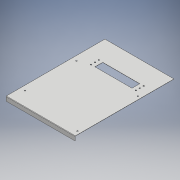
# Autodesk Inventor part: dads trunk
Saved by Autodesk Inventor 2018 (Build 220112000, 112)
## iProperties
Created: 2018-06-19
Part Number: dads trunk
Material: Generic
Document SubType Name: Sheet Metal
Designer: John Viljoen
Density: 1 g/cm^3
Flat Pattern Width: 26.3891 cm
Flat Pattern Length: 17.7174 cm
Flat Pattern Area: 467.546 cm^2
Sheet Metal Rule: Default_mm
Sheet Metal Width: 263.891 mm
Sheet Metal Length: 177.174 mm
Sheet Metal Area: 46754.619 mm^2
Appearance: Default
Author: John Viljoen
Autodesk Inventor part; units mm, degrees
ref_plane "YZ Plane" through (0, 0, 0) normal (1, 0, 0) x (0, 1, 0)
ref_plane "XZ Plane" through (0, 0, 0) normal (0, 1, 0) x (-1, 0, 0)
ref_plane "XY Plane" through (0, 0, 0) normal (0, 0, 1) x (1, 0, 0)
sketch "Sketch1" plane through (0, 0, 0) normal (0, 0, 1) x (1, 0, 0)
  line L0 (0, 0) -> (181.174, 0)
  line L1 (181.174, 0) -> (181.174, 253.26)
  line L2 (181.174, 253.26) -> (0, 253.26)
  line L3 (0, 253.26) -> (0, 0)
  dimension "d0" = 181.174
  dimension "d1" = 253.26
  measures "d0" distance of L2.end L1.end
  measures "d1" distance of L1.end L0.end
extrude "Plate1" add sketch "Sketch1" along normal blind 0.5
sketch "Sketch3" plane through (0, 0, 0.5) normal (0, 0, 1) x (1, 0, 0)
  line L0 (181.174, 253.26) -> (181.174, 0) projected
  line L1 (181.174, 253.26) -> (181.174, 168.36) construction
  line L2 (181.174, 168.36) -> (169.327, 168.36) construction
  line L3 (169.327, 168.36) -> (11.847, 168.36) construction
  line L4 (169.327, 168.36) -> (169.327, 13.48) construction
  circle A0 centre (169.327, 13.48) radius 1.5
  circle A1 centre (169.327, 168.36) radius 1.5
  circle A2 centre (11.847, 168.36) radius 1.5
  point P0 (181.174, 0.5)
  point P1 (0, 0)
  dimension "d13" = 84.9
  dimension "d14" = 11.847
  dimension "d15" = 157.48
  dimension "d16" = 154.88
  dimension "d17" = 3
  dimension "d18" = 3
  dimension "d19" = 3
  constraints: 8 end point, 3 centre point, 3 coincident, 1 horizontal, 1 perpendicular, 1 point on line, 1 vertical
  measures "d13" distance of L0.start L1.end
  measures "d14" distance of L1.end L2.end
  measures "d15" distance of L2.end L3.end
  measures "d16" distance of L2.end L4.end
  measures "d17" diameter of A0
  measures "d18" diameter of A1
  measures "d19" diameter of A2
extrude "Extrusion1" cut sketch "Sketch3" against normal blind 10
sketch "Sketch5" plane through (0, 0, 0.5) normal (0, 0, 1) x (1, 0, 0)
  circle A0 centre (11.847, 168.36) radius 1.5 projected
  line L0 (11.847, 168.36) -> (11.847, 35.808) construction
  line L1 (11.847, 168.36) -> (144.399, 168.36) construction
  line L2 (11.847, 35.808) -> (11.847, 36.34) construction
  circle A1 centre (11.847, 36.34) radius 1.5
  point P0 (0, 0)
  dimension "d28" = 90
  dimension "d32" = 0.532
  dimension "d33" = 3
  constraints: 6 end point, 2 coincident, 1 centre point, 1 horizontal, 1 perpendicular, 1 point on line
  measures "d28" angle of L0 L1
  measures "d32" distance of L2.start L2.end
  measures "d33" diameter of A1
extrude "Extrusion4" cut sketch "Sketch5" against normal blind 10 contours A1
sketch "Sketch7" plane through (0, 0, 0) normal (0, -1, 0) x (1, 0, 0)
  line L0 (181.174, 0) -> (0, 0)
  line L1 (0, 0) -> (0, -10.5)
  line L2 (0, -10.5) -> (181.174, -10.5)
  line L3 (181.174, -10.5) -> (181.174, 0)
  constraints: 6 end point, 1 horizontal, 1 perpendicular, 1 vertical
edge flange "Flange2" height 11 angle 90 thickness 0.5 bend radius 0.5 thickness toward (0, -1, 0) relief tear relief width 0.5 relief depth 0.25 edges at (90.587, 0, 0) wall of the first edge with corners at (181.174, 0, 0) (0, 0, 0) (0, 0, -10.5) (181.174, 0, -10.5)
bend "Bend2"
corner "Corner2"
sketch "Sketch8" plane through (0, 0, 0.5) normal (0, 0, 1) x (1, 0, 0)
  line L0 (181.174, 253.26) -> (0, 253.26) projected
  line L1 (181.174, 253.26) -> (177.174, 253.26)
  line L2 (177.174, 253.26) -> (177.174, -19.1311)
  line L3 (177.174, -19.1311) -> (181.174, -19.1311)
  line L4 (181.174, -19.1311) -> (181.174, 253.26)
  point P0 (0, 0)
  dimension "d46" = 4
  constraints: 8 end point, 2 parallel, 1 horizontal, 1 perpendicular
  measures "d46" distance of L3.end L2.end
extrude "Extrusion5" cut sketch "Sketch8" against normal through all
sketch "Sketch9" plane through (0, 0, 0.5) normal (0, 0, 1) x (1, 0, 0)
  line L0 (177.174, 253.26) -> (177.174, 198.82) construction
  line L1 (177.174, 253.26) -> (177.174, 0.5) construction
  line L2 (177.174, 198.82) -> (153.862, 198.82) construction
  circle A0 centre (153.862, 198.82) radius 1.5
  line L3 (153.862, 198.82) -> (153.862, 188.82) construction
  line L4 (153.862, 188.82) -> (153.862, 178.82) construction
  circle A1 centre (153.862, 188.82) radius 1.5
  circle A2 centre (153.862, 178.82) radius 1.5
  line L5 (153.862, 198.82) -> (38.862, 198.82) construction
  circle A3 centre (38.862, 198.82) radius 1.5
  circle A4 centre (38.862, 188.82) radius 1.5
  circle A5 centre (38.862, 178.82) radius 1.5
  point P0 (0, 0)
  dimension "d49" = 54.44
  dimension "d50" = 23.312
  dimension "d55" = 3
  dimension "d58" = 10
  dimension "d59" = 10
  dimension "d60" = 3
  dimension "d61" = 3
  dimension "d62" = 115
  dimension "d63" = 3
  dimension "d64" = 3
  dimension "d65" = 3
  constraints: 10 end point, 6 centre point, 4 coincident, 2 point on line, 1 horizontal, 1 perpendicular, 1 vertical
  measures "d49" distance of L0.start L0.end
  measures "d50" distance of L0.end L2.end
  measures "d55" diameter of A0
  measures "d58" distance of L3.start L3.end
  measures "d59" distance of L3.end L4.end
  measures "d60" diameter of A1
  measures "d61" diameter of A2
  measures "d62" distance of L3.start L5.end
  measures "d63" diameter of A3
  measures "d64" diameter of A4
  measures "d65" diameter of A5
extrude "Extrusion7" cut sketch "Sketch9" against normal blind 10
sketch "Sketch10" plane through (0, 0, 0.5) normal (0, 0, 1) x (1, 0, 0)
  circle A0 centre (153.862, 198.82) radius 1.5 projected
  circle A1 centre (38.862, 198.82) radius 1.5 projected
  line L0 (38.862, 198.82) -> (48.862, 198.82) construction
  line L1 (153.862, 198.82) -> (143.862, 198.82) construction
  line L2 (48.862, 198.82) -> (143.862, 198.82)
  line L3 (143.862, 198.82) -> (143.862, 178.82)
  line L4 (143.862, 178.82) -> (48.862, 178.82)
  line L5 (48.862, 178.82) -> (48.862, 198.82)
  point P0 (0, 0)
  dimension "d68" = 10
  dimension "d69" = 10
  dimension "d70" = 20
  constraints: 12 end point, 3 horizontal, 2 parallel, 1 perpendicular
  measures "d68" distance of L0.start L0.end
  measures "d69" distance of L1.start L1.end
  measures "d70" distance of L2.end L3.end
extrude "Extrusion8" cut sketch "Sketch10" against normal blind 10 contours L2 L3 L4 L5
equation "\"d2\" = Thickness"
equation "\"d36\" = BendReliefWidth"
equation "\"d37\" = BendReliefDepth"
equation "\"d38\" = MinimumRemnant"
equation "\"d39\" = TransitionRadius"
equation "\"d42\" = BendRadius"
equation "\"d43\" = CornerReliefSize"
equation "\"d44\" = GapSize"
equation "\"d45\" = JacobiRadiusSize"
equation "\"BendRadius\" = Thickness"
equation "\"BendReliefWidth\" = Thickness"
equation "\"BendReliefDepth\" = 0.5 * Thickness"
equation "\"CornerReliefSize\" = 4 * Thickness"
equation "\"MinimumRemnant\" = 2 * Thickness"
equation "\"TransitionRadius\" = BendRadius"
equation "\"JacobiRadiusSize\" = BendRadius"
equation "\"GapSize\" = Thickness"
equation "\"Thickness\" = 0.5"
body "Solid1"
